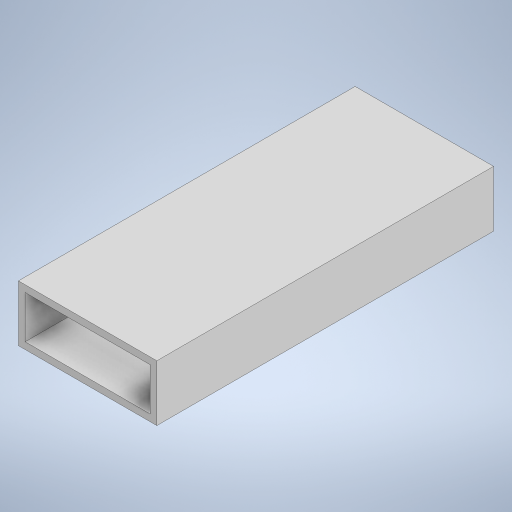
# Autodesk Inventor part: caja_grafeno
Saved by Autodesk Inventor 2024 (Build 280153000, 153)
## iProperties
Created: 2024-02-08
Part Number: caja_grafeno
Material: Genérico
Document SubType Name: Modeling
Designer: DANIELA GALEANO
Density: 1 g/cm^3
Appearance: Valor por defecto
Author: DANIELA GALEANO
Autodesk Inventor part; units mm, degrees
ref_plane "YZ Plane" through (0, 0, 0) normal (1, 0, 0) x (0, 1, 0)
ref_plane "XZ Plane" through (0, 0, 0) normal (0, 1, 0) x (-1, 0, 0)
ref_plane "XY Plane" through (0, 0, 0) normal (0, 0, 1) x (1, 0, 0)
sketch "Boceto1" plane through (0, 0, 0) normal (0, 1, 0) x (-1, 0, 0)
  line L0 (15.5342, 31.1771) -> (-21.4658, 31.1771)
  line L1 (-21.4658, 31.1771) -> (-21.4658, -58.8229)
  line L2 (-21.4658, -58.8229) -> (15.5342, -58.8229)
  line L3 (15.5342, -58.8229) -> (15.5342, 31.1771)
  point P0 (0, 0)
  dimension "d0" = 37
  dimension "d1" = 90
  constraints: 8 end point, 2 parallel, 1 horizontal, 1 perpendicular
  measures "d0" distance of L0.start L0.end
  measures "d1" distance of L2.end L0.start
extrude "Extrusión1" add sketch "Boceto1" along normal blind 15
sketch "Boceto2" plane through (-15.5342, 0, 31.1771) normal (0, 0, 1) x (1, 0, 0)
  line L0 (1.8, 13.2) -> (35.2, 13.2)
  line L1 (35.2, 13.2) -> (35.2, 1.8)
  line L2 (35.2, 1.8) -> (1.8, 1.8)
  line L3 (1.8, 1.8) -> (1.8, 13.2)
  line L4 (0, 15) -> (37, 15) projected
  line L5 (0, 0) -> (37, 0) projected
  line L6 (0, 0) -> (0, 15) projected
  line L7 (37, 0) -> (37, 15) projected
  point P0 (15.5342, 0)
  dimension "d4" = 1.8
  dimension "d5" = 1.8
  dimension "d6" = 1.8
  dimension "d7" = 1.8
  dimension "d8" = 33.4
  dimension "d9" = 11.4
  constraints: 8 end point, 2 parallel, 1 horizontal, 1 perpendicular
  measures "d4" distance between parallel lines of L4 L0
  measures "d5" distance between parallel lines of L5 L2
  measures "d6" distance between parallel lines of L6 L3
  measures "d7" distance between parallel lines of L7 L1
  measures "d8" distance of L0.start L0.end
  measures "d9" distance of L0.end L1.end
extrude "Extrusión2" cut sketch "Boceto2" against normal blind 90 contours L0 L1 L2 L3
